Autodesk Fusion 360 part; units mm, degrees
(part 3 of 4)
extrude "Foro_PCB_reale_04" cut sketch "Schizzo5 (10)" along normal blind 2 bodies 26 in component "10_Modulo_cannone_reale_PCB_solenoide_canna"
ref_plane "Piano di lavoro2" through (0, 0, 85.5) normal (0, 0, 1) x (1, 0, 0) in component "10_Modulo_cannone_reale_PCB_solenoide_canna"
sketch "Schizzo6 (8)" plane through (0, 0, 85.5) normal (0, 0, 1) x (1, 0, 0) in component "10_Modulo_cannone_reale_PCB_solenoide_canna"
  line L0 (-10, 2.5) -> (10, 2.5)
  line L1 (10, 2.5) -> (10, 27.5)
  line L2 (10, 27.5) -> (-10, 27.5)
  line L3 (-10, 27.5) -> (-10, 2.5)
extrude "Estrusione_Appoggio_solenoide_su_PCB" add sketch "Schizzo6 (8)" along normal blind 1 separate body makes body 27 in component "10_Modulo_cannone_reale_PCB_solenoide_canna"
ref_plane "Piano di lavoro3" through (0, 2.5, 0) normal (0, 1, 0) x (0, 0, 1) in component "10_Modulo_cannone_reale_PCB_solenoide_canna"
sketch "Schizzo7 (8)" plane through (0, 2.5, 0) normal (0, 1, 0) x (1, 0, 0) in component "10_Modulo_cannone_reale_PCB_solenoide_canna"
  circle A0 centre (0, -96.5) radius 10
extrude "Estrusione_Corpo_solenoide_riferimento" add sketch "Schizzo7 (8)" along normal blind 25 separate body makes body 28 in component "10_Modulo_cannone_reale_PCB_solenoide_canna"
ref_plane "Piano di lavoro4" through (0, 2.5, 0) normal (0, 1, 0) x (0, 0, 1) in component "10_Modulo_cannone_reale_PCB_solenoide_canna"
sketch "Schizzo8 (8)" plane through (0, 2.5, 0) normal (0, 1, 0) x (1, 0, 0) in component "10_Modulo_cannone_reale_PCB_solenoide_canna"
  circle A0 centre (0, -96.5) radius 5
extrude "Passaggio_canna_nel_solenoide" cut sketch "Schizzo8 (8)" along normal blind 25 bodies 28 in component "10_Modulo_cannone_reale_PCB_solenoide_canna"
ref_plane "Piano di lavoro5" through (0, 27.5, 0) normal (0, 1, 0) x (0, 0, 1) in component "10_Modulo_cannone_reale_PCB_solenoide_canna"
sketch "Schizzo9 (8)" plane through (0, 27.5, 0) normal (0, 1, 0) x (1, 0, 0) in component "10_Modulo_cannone_reale_PCB_solenoide_canna"
  circle A0 centre (0, -96.5) radius 5
extrude "Estrusione_Canna_tubolare_esterna" add sketch "Schizzo9 (8)" along normal blind 46 separate body makes body 29 in component "10_Modulo_cannone_reale_PCB_solenoide_canna"
ref_plane "Piano di lavoro6" through (0, 27.5, 0) normal (0, 1, 0) x (0, 0, 1) in component "10_Modulo_cannone_reale_PCB_solenoide_canna"
sketch "Schizzo10 (8)" plane through (0, 27.5, 0) normal (0, 1, 0) x (1, 0, 0) in component "10_Modulo_cannone_reale_PCB_solenoide_canna"
  circle A0 centre (0, -96.5) radius 4
extrude "Foro_interno_canna_tubolare" cut sketch "Schizzo10 (8)" along normal blind 46 bodies 29 in component "10_Modulo_cannone_reale_PCB_solenoide_canna"
ref_plane "Piano di lavoro1" through (0, -38, 0) normal (0, 1, 0) x (0, 0, 1) in component "11_Guscio_fisso_posteriore_torretta_removibile"
sketch "Schizzo1 (23)" plane through (0, -38, 0) normal (0, 1, 0) x (1, 0, 0) in component "11_Guscio_fisso_posteriore_torretta_removibile"
  line L0 (-43, -49.5) -> (43, -49.5)
  line L1 (43, -49.5) -> (43, -102.5)
  line L2 (43, -102.5) -> (-43, -102.5)
  line L3 (-43, -102.5) -> (-43, -49.5)
extrude "Estrusione_Parete_posteriore_guscio_torretta" add sketch "Schizzo1 (23)" along normal blind 2.5 separate body makes body 30 in component "11_Guscio_fisso_posteriore_torretta_removibile"
ref_plane "Piano di lavoro2" through (-43, 0, 0) normal (1, 0, 0) x (0, 1, 0) in component "11_Guscio_fisso_posteriore_torretta_removibile"
sketch "Schizzo2 (21)" plane through (-43, 0, 0) normal (1, 0, 0) x (0, 0, -1) in component "11_Guscio_fisso_posteriore_torretta_removibile"
  line L0 (-49.5, -38) -> (-102.5, -38)
  line L1 (-102.5, -38) -> (-102.5, -27.8)
  line L2 (-102.5, -27.8) -> (-49.5, -27.8)
  line L3 (-49.5, -27.8) -> (-49.5, -38)
extrude "Estrusione_Fianco_cofano_Sinistra" add sketch "Schizzo2 (21)" along normal blind 2.5 bodies 30 in component "11_Guscio_fisso_posteriore_torretta_removibile"
ref_plane "Piano di lavoro3" through (40.5, 0, 0) normal (1, 0, 0) x (0, 1, 0) in component "11_Guscio_fisso_posteriore_torretta_removibile"
sketch "Schizzo3 (19)" plane through (40.5, 0, 0) normal (1, 0, 0) x (0, 0, -1) in component "11_Guscio_fisso_posteriore_torretta_removibile"
  line L0 (-49.5, -38) -> (-102.5, -38)
  line L1 (-102.5, -38) -> (-102.5, -27.8)
  line L2 (-102.5, -27.8) -> (-49.5, -27.8)
  line L3 (-49.5, -27.8) -> (-49.5, -38)
extrude "Estrusione_Fianco_cofano_Destra" add sketch "Schizzo3 (19)" along normal blind 2.5 bodies 30 in component "11_Guscio_fisso_posteriore_torretta_removibile"
ref_plane "Piano di lavoro4" through (0, 0, 100) normal (0, 0, 1) x (1, 0, 0) in component "11_Guscio_fisso_posteriore_torretta_removibile"
sketch "Schizzo4 (19)" plane through (0, 0, 100) normal (0, 0, 1) x (1, 0, 0) in component "11_Guscio_fisso_posteriore_torretta_removibile"
  line L0 (-43, -38) -> (43, -38)
  line L1 (43, -38) -> (43, -27.8)
  line L2 (43, -27.8) -> (-43, -27.8)
  line L3 (-43, -27.8) -> (-43, -38)
extrude "Estrusione_Tetto_cofano_posteriore" add sketch "Schizzo4 (19)" along normal blind 2.5 bodies 30 in component "11_Guscio_fisso_posteriore_torretta_removibile"
ref_plane "Piano di lavoro5" through (-43, 0, 0) normal (1, 0, 0) x (0, 1, 0) in component "11_Guscio_fisso_posteriore_torretta_removibile"
sketch "Schizzo5 (11)" plane through (-43, 0, 0) normal (1, 0, 0) x (0, 0, -1) in component "11_Guscio_fisso_posteriore_torretta_removibile"
  circle A0 centre (-54.5, -30.3) radius 1.35
extrude "Foro_M2_5_cofano_Sinistra_01" cut sketch "Schizzo5 (11)" along normal blind 2.5 bodies 30 in component "11_Guscio_fisso_posteriore_torretta_removibile"
ref_plane "Piano di lavoro27" through (-40, 0, 0) normal (1, 0, 0) x (0, 1, 0) in component "04_Torretta_parte_fissa_azimut"
sketch "Schizzo41 (2)" plane through (-40, 0, 0) normal (1, 0, 0) x (0, 0, -1) in component "04_Torretta_parte_fissa_azimut"
  circle A0 centre (-54.5, -30.3) radius 1.1
extrude "Preforo_M2_5_cofano_telaio_Sinistra_01" cut sketch "Schizzo41 (2)" along normal blind 4 bodies 14 in component "04_Torretta_parte_fissa_azimut"
ref_plane "Piano di lavoro6" through (-43, 0, 0) normal (1, 0, 0) x (0, 1, 0) in component "11_Guscio_fisso_posteriore_torretta_removibile"
sketch "Schizzo6 (9)" plane through (-43, 0, 0) normal (1, 0, 0) x (0, 0, -1) in component "11_Guscio_fisso_posteriore_torretta_removibile"
  circle A0 centre (-94.5, -30.3) radius 1.35
extrude "Foro_M2_5_cofano_Sinistra_02" cut sketch "Schizzo6 (9)" along normal blind 2.5 bodies 30 in component "11_Guscio_fisso_posteriore_torretta_removibile"
ref_plane "Piano di lavoro28" through (-40, 0, 0) normal (1, 0, 0) x (0, 1, 0) in component "04_Torretta_parte_fissa_azimut"
sketch "Schizzo42 (2)" plane through (-40, 0, 0) normal (1, 0, 0) x (0, 0, -1) in component "04_Torretta_parte_fissa_azimut"
  circle A0 centre (-94.5, -30.3) radius 1.1
extrude "Preforo_M2_5_cofano_telaio_Sinistra_02" cut sketch "Schizzo42 (2)" along normal blind 4 bodies 14 in component "04_Torretta_parte_fissa_azimut"
ref_plane "Piano di lavoro7" through (40.5, 0, 0) normal (1, 0, 0) x (0, 1, 0) in component "11_Guscio_fisso_posteriore_torretta_removibile"
sketch "Schizzo7 (9)" plane through (40.5, 0, 0) normal (1, 0, 0) x (0, 0, -1) in component "11_Guscio_fisso_posteriore_torretta_removibile"
  circle A0 centre (-54.5, -30.3) radius 1.35
extrude "Foro_M2_5_cofano_Destra_01" cut sketch "Schizzo7 (9)" along normal blind 2.5 bodies 30 in component "11_Guscio_fisso_posteriore_torretta_removibile"
ref_plane "Piano di lavoro29" through (36, 0, 0) normal (1, 0, 0) x (0, 1, 0) in component "04_Torretta_parte_fissa_azimut"
sketch "Schizzo43 (2)" plane through (36, 0, 0) normal (1, 0, 0) x (0, 0, -1) in component "04_Torretta_parte_fissa_azimut"
  circle A0 centre (-54.5, -30.3) radius 1.1
extrude "Preforo_M2_5_cofano_telaio_Destra_01" cut sketch "Schizzo43 (2)" along normal blind 4 bodies 14 in component "04_Torretta_parte_fissa_azimut"
ref_plane "Piano di lavoro8" through (40.5, 0, 0) normal (1, 0, 0) x (0, 1, 0) in component "11_Guscio_fisso_posteriore_torretta_removibile"
sketch "Schizzo8 (9)" plane through (40.5, 0, 0) normal (1, 0, 0) x (0, 0, -1) in component "11_Guscio_fisso_posteriore_torretta_removibile"
  circle A0 centre (-94.5, -30.3) radius 1.35
extrude "Foro_M2_5_cofano_Destra_02" cut sketch "Schizzo8 (9)" along normal blind 2.5 bodies 30 in component "11_Guscio_fisso_posteriore_torretta_removibile"
ref_plane "Piano di lavoro30" through (36, 0, 0) normal (1, 0, 0) x (0, 1, 0) in component "04_Torretta_parte_fissa_azimut"
sketch "Schizzo44" plane through (36, 0, 0) normal (1, 0, 0) x (0, 0, -1) in component "04_Torretta_parte_fissa_azimut"
  circle A0 centre (-94.5, -30.3) radius 1.1
extrude "Preforo_M2_5_cofano_telaio_Destra_02" cut sketch "Schizzo44" along normal blind 4 bodies 14 in component "04_Torretta_parte_fissa_azimut"
ref_plane "Piano di lavoro1" through (-66.5, 0, 0) normal (1, 0, 0) x (0, 1, 0) in component "12_Carter_SG90_Sinistro_removibile"
sketch "Schizzo1 (24)" plane through (-66.5, 0, 0) normal (1, 0, 0) x (0, 0, -1) in component "12_Carter_SG90_Sinistro_removibile"
  line L0 (-71.9, -27.8) -> (-93.6, -27.8)
  line L1 (-93.6, -27.8) -> (-93.6, 16.5)
  line L2 (-93.6, 16.5) -> (-71.9, 16.5)
  line L3 (-71.9, 16.5) -> (-71.9, -27.8)
extrude "Estrusione_Parete_esterna_carter_Sinistro" add sketch "Schizzo1 (24)" along normal blind 2.5 separate body makes body 31 in component "12_Carter_SG90_Sinistro_removibile"
ref_plane "Piano di lavoro2" through (0, -27.8, 0) normal (0, 1, 0) x (0, 0, 1) in component "12_Carter_SG90_Sinistro_removibile"
sketch "Schizzo2 (22)" plane through (0, -27.8, 0) normal (0, 1, 0) x (1, 0, 0) in component "12_Carter_SG90_Sinistro_removibile"
  line L0 (-66.5, -71.9) -> (-40.5, -71.9)
  line L1 (-40.5, -71.9) -> (-40.5, -93.6)
  line L2 (-40.5, -93.6) -> (-66.5, -93.6)
  line L3 (-66.5, -93.6) -> (-66.5, -71.9)
extrude "Estrusione_Parete_Posteriore_carter_Sinistro" add sketch "Schizzo2 (22)" along normal blind 2.5 bodies 31 in component "12_Carter_SG90_Sinistro_removibile"
ref_plane "Piano di lavoro3" through (0, 14, 0) normal (0, 1, 0) x (0, 0, 1) in component "12_Carter_SG90_Sinistro_removibile"
sketch "Schizzo3 (20)" plane through (0, 14, 0) normal (0, 1, 0) x (1, 0, 0) in component "12_Carter_SG90_Sinistro_removibile"
  line L0 (-66.5, -71.9) -> (-40.5, -71.9)
  line L1 (-40.5, -71.9) -> (-40.5, -93.6)
  line L2 (-40.5, -93.6) -> (-66.5, -93.6)
  line L3 (-66.5, -93.6) -> (-66.5, -71.9)
extrude "Estrusione_Parete_Anteriore_carter_Sinistro" add sketch "Schizzo3 (20)" along normal blind 2.5 bodies 31 in component "12_Carter_SG90_Sinistro_removibile"
ref_plane "Piano di lavoro4" through (0, 0, 91.1) normal (0, 0, 1) x (1, 0, 0) in component "12_Carter_SG90_Sinistro_removibile"
sketch "Schizzo4 (20)" plane through (0, 0, 91.1) normal (0, 0, 1) x (1, 0, 0) in component "12_Carter_SG90_Sinistro_removibile"
  line L0 (-66.5, -27.8) -> (-40.5, -27.8)
  line L1 (-40.5, -27.8) -> (-40.5, 16.5)
  line L2 (-40.5, 16.5) -> (-66.5, 16.5)
  line L3 (-66.5, 16.5) -> (-66.5, -27.8)
extrude "Estrusione_Tetto_carter_Sinistro" add sketch "Schizzo4 (20)" along normal blind 2.5 bodies 31 in component "12_Carter_SG90_Sinistro_removibile"
ref_plane "Piano di lavoro5" through (-66.5, 0, 0) normal (1, 0, 0) x (0, 1, 0) in component "12_Carter_SG90_Sinistro_removibile"
sketch "Schizzo5 (12)" plane through (-66.5, 0, 0) normal (1, 0, 0) x (0, 0, -1) in component "12_Carter_SG90_Sinistro_removibile"
  circle A0 centre (-81.5, -23.55) radius 1.35
extrude "Foro_M2_5_carter_Sinistro_01" cut sketch "Schizzo5 (12)" along normal blind 2.5 bodies 31 in component "12_Carter_SG90_Sinistro_removibile"
ref_plane "Piano di lavoro6" through (-66.5, 0, 0) normal (1, 0, 0) x (0, 1, 0) in component "12_Carter_SG90_Sinistro_removibile"
sketch "Schizzo6 (10)" plane through (-66.5, 0, 0) normal (1, 0, 0) x (0, 0, -1) in component "12_Carter_SG90_Sinistro_removibile"
  circle A0 centre (-81.5, 12.25) radius 1.35
extrude "Foro_M2_5_carter_Sinistro_02" cut sketch "Schizzo6 (10)" along normal blind 2.5 bodies 31 in component "12_Carter_SG90_Sinistro_removibile"
ref_plane "Piano di lavoro1" through (64, 0, 0) normal (1, 0, 0) x (0, 1, 0) in component "13_Carter_SG90_Destro_removibile"
sketch "Schizzo1 (25)" plane through (64, 0, 0) normal (1, 0, 0) x (0, 0, -1) in component "13_Carter_SG90_Destro_removibile"
  line L0 (-71.9, -27.8) -> (-93.6, -27.8)
  line L1 (-93.6, -27.8) -> (-93.6, 16.5)
  line L2 (-93.6, 16.5) -> (-71.9, 16.5)
  line L3 (-71.9, 16.5) -> (-71.9, -27.8)
extrude "Estrusione_Parete_esterna_carter_Destro" add sketch "Schizzo1 (25)" along normal blind 2.5 separate body makes body 32 in component "13_Carter_SG90_Destro_removibile"
ref_plane "Piano di lavoro2" through (0, -27.8, 0) normal (0, 1, 0) x (0, 0, 1) in component "13_Carter_SG90_Destro_removibile"
sketch "Schizzo2 (23)" plane through (0, -27.8, 0) normal (0, 1, 0) x (1, 0, 0) in component "13_Carter_SG90_Destro_removibile"
  line L0 (40.5, -71.9) -> (66.5, -71.9)
  line L1 (66.5, -71.9) -> (66.5, -93.6)
  line L2 (66.5, -93.6) -> (40.5, -93.6)
  line L3 (40.5, -93.6) -> (40.5, -71.9)
extrude "Estrusione_Parete_Posteriore_carter_Destro" add sketch "Schizzo2 (23)" along normal blind 2.5 bodies 32 in component "13_Carter_SG90_Destro_removibile"
ref_plane "Piano di lavoro3" through (0, 14, 0) normal (0, 1, 0) x (0, 0, 1) in component "13_Carter_SG90_Destro_removibile"
sketch "Schizzo3 (21)" plane through (0, 14, 0) normal (0, 1, 0) x (1, 0, 0) in component "13_Carter_SG90_Destro_removibile"
  line L0 (40.5, -71.9) -> (66.5, -71.9)
  line L1 (66.5, -71.9) -> (66.5, -93.6)
  line L2 (66.5, -93.6) -> (40.5, -93.6)
  line L3 (40.5, -93.6) -> (40.5, -71.9)
extrude "Estrusione_Parete_Anteriore_carter_Destro" add sketch "Schizzo3 (21)" along normal blind 2.5 bodies 32 in component "13_Carter_SG90_Destro_removibile"
ref_plane "Piano di lavoro4" through (0, 0, 91.1) normal (0, 0, 1) x (1, 0, 0) in component "13_Carter_SG90_Destro_removibile"
sketch "Schizzo4 (21)" plane through (0, 0, 91.1) normal (0, 0, 1) x (1, 0, 0) in component "13_Carter_SG90_Destro_removibile"
  line L0 (40.5, -27.8) -> (66.5, -27.8)
  line L1 (66.5, -27.8) -> (66.5, 16.5)
  line L2 (66.5, 16.5) -> (40.5, 16.5)
  line L3 (40.5, 16.5) -> (40.5, -27.8)
extrude "Estrusione_Tetto_carter_Destro" add sketch "Schizzo4 (21)" along normal blind 2.5 bodies 32 in component "13_Carter_SG90_Destro_removibile"
ref_plane "Piano di lavoro5" through (64, 0, 0) normal (1, 0, 0) x (0, 1, 0) in component "13_Carter_SG90_Destro_removibile"
sketch "Schizzo5 (13)" plane through (64, 0, 0) normal (1, 0, 0) x (0, 0, -1) in component "13_Carter_SG90_Destro_removibile"
  circle A0 centre (-81.5, -23.55) radius 1.35
extrude "Foro_M2_5_carter_Destro_01" cut sketch "Schizzo5 (13)" along normal blind 2.5 bodies 32 in component "13_Carter_SG90_Destro_removibile"
ref_plane "Piano di lavoro6" through (64, 0, 0) normal (1, 0, 0) x (0, 1, 0) in component "13_Carter_SG90_Destro_removibile"
sketch "Schizzo6 (11)" plane through (64, 0, 0) normal (1, 0, 0) x (0, 0, -1) in component "13_Carter_SG90_Destro_removibile"
  circle A0 centre (-81.5, 12.25) radius 1.35
extrude "Foro_M2_5_carter_Destro_02" cut sketch "Schizzo6 (11)" along normal blind 2.5 bodies 32 in component "13_Carter_SG90_Destro_removibile"
ref_plane "Piano di lavoro1" through (0, 0, 83.5) normal (0, 0, 1) x (1, 0, 0) in component "14_Guscio_mobile_cannone_removibile"
sketch "Schizzo1 (26)" plane through (0, 0, 83.5) normal (0, 0, 1) x (1, 0, 0) in component "14_Guscio_mobile_cannone_removibile"
  line L0 (-28, -13) -> (-25.5, -13)
  line L1 (-25.5, -13) -> (-25.5, 43)
  line L2 (-25.5, 43) -> (-28, 43)
  line L3 (-28, 43) -> (-28, -13)
extrude "Estrusione_Parete_mobile_Ovest" add sketch "Schizzo1 (26)" along normal blind 26 separate body makes body 33 in component "14_Guscio_mobile_cannone_removibile"
sketch "Schizzo2 (24)" plane through (0, 0, 83.5) normal (0, 0, 1) x (1, 0, 0) in component "14_Guscio_mobile_cannone_removibile"
  line L0 (-28, -13) -> (28, -13)
  line L1 (28, -13) -> (28, -10.5)
  line L2 (28, -10.5) -> (-28, -10.5)
  line L3 (-28, -10.5) -> (-28, -13)
extrude "Estrusione_Parete_mobile_Posteriore" add sketch "Schizzo2 (24)" along normal blind 26 bodies 33 in component "14_Guscio_mobile_cannone_removibile"
sketch "Schizzo3 (22)" plane through (0, 0, 83.5) normal (0, 0, 1) x (1, 0, 0) in component "14_Guscio_mobile_cannone_removibile"
  line L0 (25.5, -13) -> (28, -13)
  line L1 (28, -13) -> (28, 43)
  line L2 (28, 43) -> (25.5, 43)
  line L3 (25.5, 43) -> (25.5, -13)
extrude "Estrusione_Parete_mobile_Est" add sketch "Schizzo3 (22)" along normal blind 26 bodies 33 in component "14_Guscio_mobile_cannone_removibile"
ref_plane "Piano di lavoro2" through (-28, 0, 0) normal (1, 0, 0) x (0, 1, 0) in component "14_Guscio_mobile_cannone_removibile"
sketch "Schizzo4 (22)" plane through (-28, 0, 0) normal (1, 0, 0) x (0, 0, -1) in component "14_Guscio_mobile_cannone_removibile"
  circle A0 centre (-81.5, 0) radius 17.5
extrude "Scasso_guancia_elevazione_Ovest" cut sketch "Schizzo4 (22)" along normal blind 2.5 bodies 17 in component "09_Torretta_parte_mobile_elevazione"
extrude "Estrusione6" cut sketch "Schizzo4 (22)" along normal blind 2.5 bodies 22 makes body 34 at (-31, -1.093, 68.5819) in component "09A_Guancia_cornetto_Sinistra_regolabile"
extrude "Estrusione4'" cut sketch "Schizzo4 (22)" along normal blind 2.5 bodies 33 in component "14_Guscio_mobile_cannone_removibile"
ref_plane "Piano di lavoro3" through (25.5, 0, 0) normal (1, 0, 0) x (0, 1, 0) in component "14_Guscio_mobile_cannone_removibile"
sketch "Schizzo5 (14)" plane through (25.5, 0, 0) normal (1, 0, 0) x (0, 0, -1) in component "14_Guscio_mobile_cannone_removibile"
  circle A0 centre (-81.5, 0) radius 17.5
extrude "Scasso_guancia_elevazione_Est" cut sketch "Schizzo5 (14)" along normal blind 2.5 bodies 17 in component "09_Torretta_parte_mobile_elevazione"
extrude "Estrusione6'" cut sketch "Schizzo5 (14)" along normal blind 2.5 bodies 24 makes body 35 at (23.3333, -2.85, 79.5) in component "09B_Guancia_cornetto_Destra_regolabile"
extrude "Estrusione5" cut sketch "Schizzo5 (14)" along normal blind 2.5 bodies 33 in component "14_Guscio_mobile_cannone_removibile"
ref_plane "Piano di lavoro4" through (0, 0, 107) normal (0, 0, 1) x (1, 0, 0) in component "14_Guscio_mobile_cannone_removibile"
sketch "Schizzo6 (12)" plane through (0, 0, 107) normal (0, 0, 1) x (1, 0, 0) in component "14_Guscio_mobile_cannone_removibile"
  line L0 (-28, -13) -> (28, -13)
  line L1 (28, -13) -> (28, 43)
  line L2 (28, 43) -> (-28, 43)
  line L3 (-28, 43) -> (-28, -13)
extrude "Estrusione_Tetto_guscio_mobile_cannone" add sketch "Schizzo6 (12)" along normal blind 2.5 bodies 33 in component "14_Guscio_mobile_cannone_removibile"
ref_plane "Piano di lavoro5" through (0, 0, 106.2) normal (0, 0, 1) x (1, 0, 0) in component "14_Guscio_mobile_cannone_removibile"
sketch "Schizzo7 (10)" plane through (0, 0, 106.2) normal (0, 0, 1) x (1, 0, 0) in component "14_Guscio_mobile_cannone_removibile"
  line L0 (-15, -13) -> (-7, -13)
  line L1 (-7, -13) -> (-7, 2)
  line L2 (-7, 2) -> (-15, 2)
  line L3 (-15, 2) -> (-15, -13)
extrude "Estrusione_Longherone_rinforzo_tasca_culatta_Ovest" add sketch "Schizzo7 (10)" along normal blind 1 bodies 33 in component "14_Guscio_mobile_cannone_removibile"
sketch "Schizzo8 (10)" plane through (0, 0, 106.2) normal (0, 0, 1) x (1, 0, 0) in component "14_Guscio_mobile_cannone_removibile"
  line L0 (7, -13) -> (15, -13)
  line L1 (15, -13) -> (15, 2)
  line L2 (15, 2) -> (7, 2)
  line L3 (7, 2) -> (7, -13)
extrude "Estrusione_Longherone_rinforzo_tasca_culatta_Est" add sketch "Schizzo8 (10)" along normal blind 1 bodies 33 in component "14_Guscio_mobile_cannone_removibile"
sketch "Schizzo9 (9)" plane through (0, 0, 106.2) normal (0, 0, 1) x (1, 0, 0) in component "14_Guscio_mobile_cannone_removibile"
  line L0 (-15, -1) -> (15, -1)
  line L1 (15, -1) -> (15, 2)
  line L2 (15, 2) -> (-15, 2)
  line L3 (-15, 2) -> (-15, -1)
extrude "Estrusione_Traversa_anteriore_rinforzo_tasca_culatta" add sketch "Schizzo9 (9)" along normal blind 1 bodies 33 in component "14_Guscio_mobile_cannone_removibile"
ref_plane "Piano di lavoro6" through (0, -13, 0) normal (0, 1, 0) x (0, 0, 1) in component "14_Guscio_mobile_cannone_removibile"
sketch "Schizzo10 (9)" plane through (0, -13, 0) normal (0, 1, 0) x (1, 0, 0) in component "14_Guscio_mobile_cannone_removibile"
  line L0 (-7, -90.5) -> (7, -90.5)
  line L1 (7, -90.5) -> (7, -109.5)
  line L2 (7, -109.5) -> (-7, -109.5)
  line L3 (-7, -109.5) -> (-7, -90.5)
extrude "Finestra_posteriore_culatta_manuale" cut sketch "Schizzo10 (9)" along normal blind 2.5 bodies 33 in component "14_Guscio_mobile_cannone_removibile"
sketch "Schizzo11 (8)" plane through (0, 0, 107) normal (0, 0, 1) x (1, 0, 0) in component "14_Guscio_mobile_cannone_removibile"
  line L0 (-7, -13) -> (7, -13)
  line L1 (7, -13) -> (7, -1)
  line L2 (7, -1) -> (-7, -1)
  line L3 (-7, -1) -> (-7, -13)
extrude "Asola_tetto_accesso_culatta_manuale" cut sketch "Schizzo11 (8)" along normal blind 2.5 bodies 33 in component "14_Guscio_mobile_cannone_removibile"
ref_plane "Piano di lavoro7" through (0, 0, 107.5) normal (0, 0, 1) x (1, 0, 0) in component "14_Guscio_mobile_cannone_removibile"
sketch "Schizzo12 (7)" plane through (0, 0, 107.5) normal (0, 0, 1) x (1, 0, 0) in component "14_Guscio_mobile_cannone_removibile"
  line L0 (-15, -13) -> (15, -13)
  line L1 (15, -13) -> (15, 2)
  line L2 (15, 2) -> (-15, 2)
  line L3 (-15, 2) -> (-15, -13)
extrude "Tasca_coperchio_culatta_a_filo" cut sketch "Schizzo12 (7)" along normal blind 2 bodies 33 in component "14_Guscio_mobile_cannone_removibile"
ref_plane "Piano di lavoro8" through (0, -6, 0) normal (0, 1, 0) x (0, 0, 1) in component "14_Guscio_mobile_cannone_removibile"
sketch "Schizzo13 (7)" plane through (0, -6, 0) normal (0, 1, 0) x (1, 0, 0) in component "14_Guscio_mobile_cannone_removibile"
  circle A0 centre (0, -96.5) radius 5.5
extrude "Estrusione_Guida_interna_culatta_manuale" add sketch "Schizzo13 (7)" along normal blind 8 separate body makes body 36 in component "14_Guscio_mobile_cannone_removibile"
ref_plane "Piano di lavoro9" through (0, -6, 0) normal (0, 1, 0) x (0, 0, 1) in component "14_Guscio_mobile_cannone_removibile"
sketch "Schizzo14 (6)" plane through (0, -6, 0) normal (0, 1, 0) x (1, 0, 0) in component "14_Guscio_mobile_cannone_removibile"
  circle A0 centre (0, -96.5) radius 4
extrude "Foro_coassiale_guida_culatta_manuale" cut sketch "Schizzo14 (6)" along normal blind 8 bodies 36 in component "14_Guscio_mobile_cannone_removibile"
ref_plane "Piano di lavoro10" through (0, 0, 100.8) normal (0, 0, 1) x (1, 0, 0) in component "14_Guscio_mobile_cannone_removibile"
sketch "Schizzo15 (6)" plane through (0, 0, 100.8) normal (0, 0, 1) x (1, 0, 0) in component "14_Guscio_mobile_cannone_removibile"
  line L0 (-2, -6) -> (2, -6)
  line L1 (2, -6) -> (2, 2)
  line L2 (2, 2) -> (-2, 2)
  line L3 (-2, 2) -> (-2, -6)
extrude "Estrusione_Nervatura_tetto_guida_culatta" add sketch "Schizzo15 (6)" along normal blind 6.4 bodies 33 36 in component "14_Guscio_mobile_cannone_removibile"
ref_plane "Piano di lavoro11" through (0, 0, 103) normal (0, 0, 1) x (1, 0, 0) in component "14_Guscio_mobile_cannone_removibile"
sketch "Schizzo16 (6)" plane through (0, 0, 103) normal (0, 0, 1) x (1, 0, 0) in component "14_Guscio_mobile_cannone_removibile"
  circle A0 centre (-10.75, -4) radius 3
extrude "Estrusione_Boss_M2_5_coperchio_culatta_01" add sketch "Schizzo16 (6)" along normal blind 4.2 bodies 33 in component "14_Guscio_mobile_cannone_removibile"
sketch "Schizzo17 (5)" plane through (0, 0, 103) normal (0, 0, 1) x (1, 0, 0) in component "14_Guscio_mobile_cannone_removibile"
  circle A0 centre (-10.75, -4) radius 1.1
extrude "Preforo_M2_5_coperchio_culatta_01" cut sketch "Schizzo17 (5)" along normal blind 4.6 bodies 33 in component "14_Guscio_mobile_cannone_removibile"
sketch "Schizzo18 (5)" plane through (0, 0, 103) normal (0, 0, 1) x (1, 0, 0) in component "14_Guscio_mobile_cannone_removibile"
  circle A0 centre (10.75, -4) radius 3
extrude "Estrusione_Boss_M2_5_coperchio_culatta_02" add sketch "Schizzo18 (5)" along normal blind 4.2 bodies 33 in component "14_Guscio_mobile_cannone_removibile"
sketch "Schizzo19 (4)" plane through (0, 0, 103) normal (0, 0, 1) x (1, 0, 0) in component "14_Guscio_mobile_cannone_removibile"
  circle A0 centre (10.75, -4) radius 1.1
extrude "Preforo_M2_5_coperchio_culatta_02" cut sketch "Schizzo19 (4)" along normal blind 4.6 bodies 33 in component "14_Guscio_mobile_cannone_removibile"
sketch "Schizzo20 (4)" plane through (0, 0, 83.5) normal (0, 0, 1) x (1, 0, 0) in component "14_Guscio_mobile_cannone_removibile"
  line L0 (-28, 40.5) -> (-5.5, 40.5)
  line L1 (-5.5, 40.5) -> (-5.5, 43)
  line L2 (-5.5, 43) -> (-28, 43)
  line L3 (-28, 43) -> (-28, 40.5)
extrude "Estrusione_Parete_mobile_Anteriore_Ovest" add sketch "Schizzo20 (4)" along normal blind 26 bodies 33 in component "14_Guscio_mobile_cannone_removibile"
sketch "Schizzo21 (4)" plane through (0, 0, 83.5) normal (0, 0, 1) x (1, 0, 0) in component "14_Guscio_mobile_cannone_removibile"
  line L0 (5.5, 40.5) -> (28, 40.5)
  line L1 (28, 40.5) -> (28, 43)
  line L2 (28, 43) -> (5.5, 43)
  line L3 (5.5, 43) -> (5.5, 40.5)
extrude "Estrusione_Parete_mobile_Anteriore_Est" add sketch "Schizzo21 (4)" along normal blind 26 bodies 33 in component "14_Guscio_mobile_cannone_removibile"
ref_plane "Piano di lavoro12" through (0, 0, 102) normal (0, 0, 1) x (1, 0, 0) in component "14_Guscio_mobile_cannone_removibile"
sketch "Schizzo22 (4)" plane through (0, 0, 102) normal (0, 0, 1) x (1, 0, 0) in component "14_Guscio_mobile_cannone_removibile"
  line L0 (-5.5, 40.5) -> (5.5, 40.5)
  line L1 (5.5, 40.5) -> (5.5, 43)
  line L2 (5.5, 43) -> (-5.5, 43)
  line L3 (-5.5, 43) -> (-5.5, 40.5)
extrude "Estrusione_Ponte_superiore_cava_U_canna" add sketch "Schizzo22 (4)" along normal blind 7.5 bodies 33 in component "14_Guscio_mobile_cannone_removibile"
ref_plane "Piano di lavoro13" through (0, -13, 0) normal (0, 1, 0) x (0, 0, 1) in component "14_Guscio_mobile_cannone_removibile"
sketch "Schizzo23 (3)" plane through (0, -13, 0) normal (0, 1, 0) x (1, 0, 0) in component "14_Guscio_mobile_cannone_removibile"
  line L0 (-3, -83.5) -> (3, -83.5)
  line L1 (3, -83.5) -> (3, -87.5)
  line L2 (3, -87.5) -> (-3, -87.5)
  line L3 (-3, -87.5) -> (-3, -83.5)
extrude "Tacca_posteriore_cavo_cannone_aperta_inferiormente" cut sketch "Schizzo23 (3)" along normal blind 2.5 bodies 33 in component "14_Guscio_mobile_cannone_removibile"
ref_plane "Piano di lavoro14" through (0, 0, 85.5) normal (0, 0, 1) x (1, 0, 0) in component "14_Guscio_mobile_cannone_removibile"
sketch "Schizzo24 (3)" plane through (0, 0, 85.5) normal (0, 0, 1) x (1, 0, 0) in component "14_Guscio_mobile_cannone_removibile"
  circle A0 centre (-20, -5) radius 5
extrude "Estrusione_Colonna_M3_guscio_mobile_01" add sketch "Schizzo24 (3)" along normal blind 21.7 bodies 33 in component "14_Guscio_mobile_cannone_removibile"
sketch "Schizzo25 (3)" plane through (0, 0, 85.5) normal (0, 0, 1) x (1, 0, 0) in component "14_Guscio_mobile_cannone_removibile"
  circle A0 centre (-20, -5) radius 1.75
extrude "Foro_M3_guscio_mobile_01" cut sketch "Schizzo25 (3)" along normal blind 24 bodies 33 in component "14_Guscio_mobile_cannone_removibile"
sketch "Schizzo26 (3)" plane through (0, 0, 85.5) normal (0, 0, 1) x (1, 0, 0) in component "14_Guscio_mobile_cannone_removibile"
  circle A0 centre (20, -5) radius 5
extrude "Estrusione_Colonna_M3_guscio_mobile_02" add sketch "Schizzo26 (3)" along normal blind 21.7 bodies 33 in component "14_Guscio_mobile_cannone_removibile"
sketch "Schizzo27 (3)" plane through (0, 0, 85.5) normal (0, 0, 1) x (1, 0, 0) in component "14_Guscio_mobile_cannone_removibile"
  circle A0 centre (20, -5) radius 1.75
extrude "Foro_M3_guscio_mobile_02" cut sketch "Schizzo27 (3)" along normal blind 24 bodies 33 in component "14_Guscio_mobile_cannone_removibile"
sketch "Schizzo28 (3)" plane through (0, 0, 85.5) normal (0, 0, 1) x (1, 0, 0) in component "14_Guscio_mobile_cannone_removibile"
  circle A0 centre (-20, 35) radius 5
extrude "Estrusione_Colonna_M3_guscio_mobile_03" add sketch "Schizzo28 (3)" along normal blind 21.7 bodies 33 in component "14_Guscio_mobile_cannone_removibile"
sketch "Schizzo29 (3)" plane through (0, 0, 85.5) normal (0, 0, 1) x (1, 0, 0) in component "14_Guscio_mobile_cannone_removibile"
  circle A0 centre (-20, 35) radius 1.75
extrude "Foro_M3_guscio_mobile_03" cut sketch "Schizzo29 (3)" along normal blind 24 bodies 33 in component "14_Guscio_mobile_cannone_removibile"
sketch "Schizzo30 (3)" plane through (0, 0, 85.5) normal (0, 0, 1) x (1, 0, 0) in component "14_Guscio_mobile_cannone_removibile"
  circle A0 centre (20, 35) radius 5
extrude "Estrusione_Colonna_M3_guscio_mobile_04" add sketch "Schizzo30 (3)" along normal blind 21.7 bodies 33 in component "14_Guscio_mobile_cannone_removibile"
sketch "Schizzo31 (3)" plane through (0, 0, 85.5) normal (0, 0, 1) x (1, 0, 0) in component "14_Guscio_mobile_cannone_removibile"
  circle A0 centre (20, 35) radius 1.75
extrude "Foro_M3_guscio_mobile_04" cut sketch "Schizzo31 (3)" along normal blind 24 bodies 33 in component "14_Guscio_mobile_cannone_removibile"
ref_plane "Piano di lavoro1" through (0, 0, 107.5) normal (0, 0, 1) x (1, 0, 0) in component "15_Coperchio_culatta_L_removibile_M2_5"
sketch "Schizzo1 (27)" plane through (0, 0, 107.5) normal (0, 0, 1) x (1, 0, 0) in component "15_Coperchio_culatta_L_removibile_M2_5"
  line L0 (-14.7, -12.7) -> (14.7, -12.7)
  line L1 (14.7, -12.7) -> (14.7, 1.7)
  line L2 (14.7, 1.7) -> (-14.7, 1.7)
  line L3 (-14.7, 1.7) -> (-14.7, -12.7)
extrude "Estrusione_Piastra_superiore_coperchio_culatta_a_filo" add sketch "Schizzo1 (27)" along normal blind 1.8 separate body makes body 37 in component "15_Coperchio_culatta_L_removibile_M2_5"
ref_plane "Piano di lavoro2" through (0, -12.7, 0) normal (0, 1, 0) x (0, 0, 1) in component "15_Coperchio_culatta_L_removibile_M2_5"
sketch "Schizzo2 (25)" plane through (0, -12.7, 0) normal (0, 1, 0) x (1, 0, 0) in component "15_Coperchio_culatta_L_removibile_M2_5"
  line L0 (-6.7, -90.8) -> (6.7, -90.8)
  line L1 (6.7, -90.8) -> (6.7, -109.2)
  line L2 (6.7, -109.2) -> (-6.7, -109.2)
  line L3 (-6.7, -109.2) -> (-6.7, -90.8)
extrude "Estrusione_Piastra_posteriore_coperchio_culatta" add sketch "Schizzo2 (25)" along normal blind 1.9 bodies 37 in component "15_Coperchio_culatta_L_removibile_M2_5"
ref_plane "Piano di lavoro3" through (0, 0, 108.1) normal (0, 0, 1) x (1, 0, 0) in component "15_Coperchio_culatta_L_removibile_M2_5"
ref_plane "Piano di lavoro4" through (0, 0, 109.3) normal (0, 0, 1) x (1, 0, 0) in component "15_Coperchio_culatta_L_removibile_M2_5"
sketch "Schizzo3 (23)" plane through (0, 0, 107.5) normal (0, 0, 1) x (1, 0, 0) in component "15_Coperchio_culatta_L_removibile_M2_5"
  circle A0 centre (-10.75, -4) radius 1.35
extrude "Foro_M2_5_coperchio_culatta_01" cut sketch "Schizzo3 (23)" along normal blind 1.8 bodies 37 in component "15_Coperchio_culatta_L_removibile_M2_5"
sketch "Schizzo4 (23)" plane through (0, 0, 108.1) normal (0, 0, 1) x (1, 0, 0) in component "15_Coperchio_culatta_L_removibile_M2_5"
  circle A0 centre (-10.75, -4) radius 1.35
sketch "Schizzo5 (15)" plane through (0, 0, 109.3) normal (0, 0, 1) x (1, 0, 0) in component "15_Coperchio_culatta_L_removibile_M2_5"
  circle A0 centre (-10.75, -4) radius 2.5
loft "Svasatura_M2_5_coperchio_culatta_01" cut profiles "Schizzo4 (23)", "Schizzo5 (15)" section 1 section 2 bodies 37 in component "15_Coperchio_culatta_L_removibile_M2_5"
sketch "Schizzo6 (13)" plane through (0, 0, 107.5) normal (0, 0, 1) x (1, 0, 0) in component "15_Coperchio_culatta_L_removibile_M2_5"
  circle A0 centre (10.75, -4) radius 1.35
extrude "Foro_M2_5_coperchio_culatta_02" cut sketch "Schizzo6 (13)" along normal blind 1.8 bodies 37 in component "15_Coperchio_culatta_L_removibile_M2_5"
sketch "Schizzo7 (11)" plane through (0, 0, 108.1) normal (0, 0, 1) x (1, 0, 0) in component "15_Coperchio_culatta_L_removibile_M2_5"
  circle A0 centre (10.75, -4) radius 1.35
sketch "Schizzo8 (11)" plane through (0, 0, 109.3) normal (0, 0, 1) x (1, 0, 0) in component "15_Coperchio_culatta_L_removibile_M2_5"
  circle A0 centre (10.75, -4) radius 2.5
loft "Svasatura_M2_5_coperchio_culatta_02" cut profiles "Schizzo7 (11)", "Schizzo8 (11)" section 1 section 2 bodies 37 in component "15_Coperchio_culatta_L_removibile_M2_5"
sketch "Schizzo1 (28)" plane through (0, 0, 0) normal (0, 1, 0) x (1, 0, 0) in component "06_Sottoassieme_coperchio_stepper_torretta"
  line L0 (0, -20) -> (0, 20)
ref_plane "Piano di lavoro1" through (0, 0, 81.5) normal (0, 0, 1) x (1, 0, 0) in component "06_Sottoassieme_coperchio_stepper_torretta"
sketch "Schizzo2 (26)" plane through (0, 0, 81.5) normal (0, 0, 1) x (1, 0, 0) in component "06_Sottoassieme_coperchio_stepper_torretta"
  line L0 (-20, 0) -> (20, 0)
component "01_Piano_inferiore_colonnine_M3_supporto_batteria_integrato" placed x (1, 0, 0) y (0, 1, 0) z (0, 0, 1) at (0, 0, 0)
component "02_Piano_superiore" placed x (1, 0, 0) y (0, 1, 0) z (0, 0, 1) at (0, 0, 0)
component "03_Guscio_laterale_continuo_carro" placed x (1, 0, 0) y (0, 1, 0) z (0, 0, 1) at (0, 0, 0)
component "05_Arduino_UNO_R4_WiFi_RIFERIMENTO_XY_quota_Z_da_definire" placed x (1, 0, 0) y (0, 1, 0) z (0, 0, 1) at (33.33, 45.71, 3)
component "06_Sottoassieme_coperchio_stepper_torretta" placed x (1, 0, 0) y (0, 1, 0) z (0, 0, 1) at (0, 0, 46)
component "01_Tetto_elettronica_removibile" placed x (1, 0, 0) y (0, 1, 0) z (0, 0, 1) at (0, 0, 0) in component "06_Sottoassieme_coperchio_stepper_torretta"
component "02A_Rondella_assiale_torretta_sostituibile" placed x (1, 0, 0) y (0, 1, 0) z (0, 0, 1) at (0, 0, 0) in component "06_Sottoassieme_coperchio_stepper_torretta"
component "02_Stepper_28BYJ48_statore_fisso_riferimento" placed x (1, 0, 0) y (0, 1, 0) z (0, 0, 1) at (0, 0, 0) in component "06_Sottoassieme_coperchio_stepper_torretta"
component "02B_Rotore_albero_28BYJ48_riferimento" placed x (1, 0, 0) y (0, 1, 0) z (0, 0, 1) at (0, 0, 0) in component "06_Sottoassieme_coperchio_stepper_torretta"
component "03_Base_rotante_D100_sede_D_stepper" placed x (1, 0, 0) y (0, 1, 0) z (0, 0, 1) at (0, 0, 0) in component "06_Sottoassieme_coperchio_stepper_torretta"
component "03A_Fermaglio_anti_sollevamento_Est_M3" placed x (1, 0, 0) y (0, 1, 0) z (0, 0, 1) at (0, 0, 0) in component "06_Sottoassieme_coperchio_stepper_torretta"
component "03A_Fermaglio_anti_sollevamento_Ovest_M3" placed x (1, 0, 0) y (0, 1, 0) z (0, 0, 1) at (0, 0, 0) in component "06_Sottoassieme_coperchio_stepper_torretta"
component "03A_Fermaglio_anti_sollevamento_Nord_M3" placed x (1, 0, 0) y (0, 1, 0) z (0, 0, 1) at (0, 0, 0) in component "06_Sottoassieme_coperchio_stepper_torretta"
component "03A_Fermaglio_anti_sollevamento_Sud_M3" placed x (1, 0, 0) y (0, 1, 0) z (0, 0, 1) at (0, 0, 0) in component "06_Sottoassieme_coperchio_stepper_torretta"
component "04_Torretta_parte_fissa_azimut" placed x (1, 0, 0) y (0, 1, 0) z (0, 0, 1) at (0, 0, 0) in component "06_Sottoassieme_coperchio_stepper_torretta"
component "05_Servo_TowerPro_SG90_Sinistro_statore_riferimento" placed x (1, 0, 0) y (0, 1, 0) z (0, 0, 1) at (0, 0, 0) in component "06_Sottoassieme_coperchio_stepper_torretta"
component "06_Servo_TowerPro_SG90_Destro_statore_riferimento" placed x (1, 0, 0) y (0, 1, 0) z (0, 0, 1) at (0, 0, 0) in component "06_Sottoassieme_coperchio_stepper_torretta"
component "09_Torretta_parte_mobile_elevazione" placed x (1, 0, 0) y (0, 1, 0) z (0, 0, 1) at (0, 0, 0) in component "06_Sottoassieme_coperchio_stepper_torretta"
component "07_Albero_e_cornetto_croce_SG90_Sinistro_riferimento" placed x (1, 0, 0) y (0, 1, 0) z (0, 0, 1) at (0, 0, 0) in component "06_Sottoassieme_coperchio_stepper_torretta"
component "08_Albero_e_cornetto_croce_SG90_Destro_riferimento" placed x (1, 0, 0) y (0, 1, 0) z (0, 0, 1) at (0, 0, 0) in component "06_Sottoassieme_coperchio_stepper_torretta"
component "09A_Guancia_cornetto_Sinistra_regolabile" placed x (1, 0, 0) y (0, 1, 0) z (0, 0, 1) at (0, 0, 0) in component "06_Sottoassieme_coperchio_stepper_torretta"
component "09B_Guancia_cornetto_Destra_regolabile" placed x (1, 0, 0) y (0, 1, 0) z (0, 0, 1) at (0, 0, 0) in component "06_Sottoassieme_coperchio_stepper_torretta"
component "10_Modulo_cannone_reale_PCB_solenoide_canna" placed x (1, 0, 0) y (0, 1, 0) z (0, 0, 1) at (0, 0, 0) in component "06_Sottoassieme_coperchio_stepper_torretta"
component "11_Guscio_fisso_posteriore_torretta_removibile" placed x (1, 0, 0) y (0, 1, 0) z (0, 0, 1) at (0, 0, 0) in component "06_Sottoassieme_coperchio_stepper_torretta"
component "12_Carter_SG90_Sinistro_removibile" placed x (1, 0, 0) y (0, 1, 0) z (0, 0, 1) at (0, 0, 0) in component "06_Sottoassieme_coperchio_stepper_torretta"
component "13_Carter_SG90_Destro_removibile" placed x (1, 0, 0) y (0, 1, 0) z (0, 0, 1) at (0, 0, 0) in component "06_Sottoassieme_coperchio_stepper_torretta"
component "14_Guscio_mobile_cannone_removibile" placed x (1, 0, 0) y (0, 1, 0) z (0, 0, 1) at (0, 0, 0) in component "06_Sottoassieme_coperchio_stepper_torretta"
component "15_Coperchio_culatta_L_removibile_M2_5" placed x (1, 0, 0) y (0, 1, 0) z (0, 0, 1) at (0, 0, 0) in component "06_Sottoassieme_coperchio_stepper_torretta"
equation "piano_inf_lunghezza = 170.0 mm" comment "Piano inferiore"
equation "piano_inf_larghezza = 160.0 mm" comment "Piano inferiore"
equation "piano_inf_spessore = 3.0 mm" comment "Piano inferiore"
equation "d4 = piano_inf_spessore"
equation "distanza_piani = 40.0 mm" comment "Luce libera fra i piani"
equation "piano_sup_lunghezza = 170.0 mm" comment "Piano superiore"
equation "piano_sup_larghezza = 160.0 mm" comment "Piano superiore"
equation "piano_sup_spessore = 3.0 mm" comment "Piano superiore"
equation "colonnina_diametro = 10.0 mm" comment "Colonnine base"
equation "foro_vite_M3 = 3.2 mm" comment "Gioco vite M3"
equation "colonnina_offset_bordo = 12.0 mm" comment "Centro colonnina dal bordo"
equation "dado_M3_chiave = 5.8 mm" comment "Sede esagonale dado M3"
equation "dado_M3_profondita = 2.6 mm" comment "Profondita sede dado M3"
equation "d15 = piano_inf_spessore + distanza_piani"
equation "d17 = piano_sup_spessore"
equation "d19 = piano_inf_spessore"
equation "d21 = piano_inf_spessore + distanza_piani - dado_M3_profondita"
equation "asola_fascetta_lunghezza = 10.0 mm" comment "Asola fascetta, asse Est-Ovest"
equation "asola_fascetta_larghezza = 5.0 mm" comment "Asola fascetta, asse Sud-Nord"
equation "d25 = piano_inf_spessore"
equation "d27 = piano_inf_spessore"
equation "d29 = piano_inf_spessore"
equation "d31 = piano_inf_spessore"
equation "foro_servizio_inferiore_larghezza = 10.0 mm" comment "Foro 10x10 vicino Arduino"
equation "foro_servizio_inferiore_lunghezza = 10.0 mm" comment "Foro 10x10 vicino Arduino"
equation "foro_servizio_inferiore_centro_x = -0.5 mm" comment "Centro quasi sull'asse del carro"
equation "foro_servizio_inferiore_da_sud = 110.0 mm" comment "20 mm oltre il centro dell'ultima asola fascetta"
equation "d37 = piano_inf_spessore"
equation "d39 = piano_sup_spessore"
equation "d41 = distanza_piani"
equation "d43 = piano_inf_spessore + distanza_piani"
equation "d45 = dado_M3_profondita"
equation "d47 = piano_sup_spessore"
equation "d49 = distanza_piani"
equation "d51 = piano_inf_spessore + distanza_piani"
equation "d53 = dado_M3_profondita"
equation "d55 = piano_sup_spessore"
equation "d57 = distanza_piani"
equation "d59 = piano_inf_spessore + distanza_piani"
equation "d61 = dado_M3_profondita"
equation "d63 = piano_sup_spessore"
equation "d65 = distanza_piani"
equation "d67 = piano_inf_spessore + distanza_piani"
equation "d69 = dado_M3_profondita"
equation "apertura_arduino_larghezza = 25.0 mm" comment "Apertura superiore sopra Arduino"
equation "apertura_arduino_lunghezza = 25.0 mm" comment "Apertura superiore sopra Arduino"
equation "apertura_arduino_centro_x = 33.33 mm" comment "Centro Est-Ovest apertura Arduino"
equation "apertura_arduino_centro_y = 45.71 mm" comment "Centro Sud-Nord apertura Arduino"
equation "apertura_pacco_batteria_larghezza = 33.0 mm" comment "Apertura superiore pacco batteria PCB cannone"
equation "apertura_pacco_batteria_lunghezza = 60.0 mm" comment "Apertura superiore pacco batteria PCB cannone"
equation "apertura_pacco_batteria_centro_x = -52.5 mm" comment "Centro Est-Ovest apertura pacco batteria PCB cannone"
equation "apertura_pacco_batteria_centro_y = -15.0 mm" comment "Centro Sud-Nord apertura pacco batteria PCB cannone"
equation "d79 = piano_sup_spessore"
equation "d81 = piano_sup_spessore"
equation "foro_piano_superiore_M2_5_guscio = 2.7 mm" comment "Quattro viti M2.5x8 per trattenere il guscio inferiore"
equation "d84 = piano_sup_spessore"
equation "d86 = piano_sup_spessore"
equation "d88 = piano_sup_spessore"
equation "d90 = piano_sup_spessore"
equation "batt_vano_lunghezza = 95.0 mm" comment "Vano batteria"
equation "batt_vano_larghezza = 40.0 mm" comment "Vano batteria"
equation "batt_esterno_lunghezza = 100.0 mm" comment "Supporto batteria"
equation "batt_esterno_larghezza = 45.0 mm" comment "Supporto batteria"
equation "batt_parete_spessore = 2.5 mm" comment "Pareti laterali"
equation "batt_parete_altezza = 17.0 mm" comment "Pareti laterali"
equation "batt_apertura_cavi = 10.0 mm" comment "Passaggio cavi"
equation "d99 = piano_inf_spessore"
equation "d101 = batt_parete_altezza"
equation "d103 = batt_parete_altezza"
equation "d105 = batt_parete_altezza"
equation "d107 = batt_parete_altezza"
equation "guscio_carro_larghezza_interna = 161.0 mm" comment "Vano interno guscio carro"
equation "guscio_carro_lunghezza_interna = 171.0 mm" comment "Vano interno guscio carro"
equation "guscio_carro_larghezza_esterna = 166.0 mm" comment "Ingombro esterno guscio carro"
equation "guscio_carro_lunghezza_esterna = 176.0 mm" comment "Ingombro esterno guscio carro"
equation "guscio_carro_parete = 2.5 mm" comment "Pareti guscio removibile"
equation "guscio_carro_altezza_inferiore = 46.0 mm" comment "Da piano inferiore a sommità piano superiore"
equation "guscio_carro_gioco_lato = 0.5 mm" comment "Gioco per lato rispetto ai piani"
equation "guscio_carro_altezza_laterale_continua = 76.0 mm" comment "Parete unica senza giunzione intermedia"
equation "guscio_linguetta_M2_5_spessore = 5.0 mm" comment "Fissaggio guscio sotto il piano superiore"
equation "guscio_linguetta_M2_5_span = 14.0 mm" comment "Fissaggio guscio sotto il piano superiore"
equation "guscio_linguetta_M2_5_profondita = 13.0 mm" comment "Fissaggio guscio sotto il piano superiore"
equation "guscio_linguetta_M2_5_preforo = 2.2 mm" comment "Preforo per M2.5x8"
equation "griglia_feritoie_per_parete = 3.0 mm" comment "Numero ridotto di feritoie fronte e retro"
equation "griglia_feritoia_larghezza = 42.0 mm" comment "Ventilazione vano inferiore"
equation "griglia_feritoia_altezza = 4.0 mm" comment "Ventilazione vano inferiore"
equation "griglia_feritoia_passo_verticale = 8.0 mm" comment "Ventilazione vano inferiore"
equation "d125 = guscio_carro_altezza_laterale_continua"
equation "d127 = guscio_carro_altezza_laterale_continua"
equation "d129 = guscio_carro_altezza_laterale_continua"
equation "d131 = guscio_carro_altezza_laterale_continua"
equation "arduino_r4_lunghezza = 68.58 mm" comment "Profilo ufficiale Arduino UNO R4 WiFi"
equation "arduino_r4_larghezza = 53.34 mm" comment "Profilo ufficiale Arduino UNO R4 WiFi"
equation "arduino_r4_spessore_pcb = 1.0 mm" comment "Spessore PCB ufficiale; quota Z di montaggio non ancora definita"
equation "arduino_r4_rotazione = 90.0 deg" comment "Jack DC orientato verso Sud"
equation "arduino_r4_centro_x = 33.33 mm" comment "Posizione planimetrica Arduino"
equation "arduino_r4_centro_y = 45.71 mm" comment "Posizione planimetrica Arduino"
equation "cop_lunghezza = 176.0 mm" comment "Ingombro coperchio"
equation "cop_larghezza = 166.0 mm" comment "Ingombro coperchio"
equation "cop_parete_altezza = 30.0 mm" comment "Quota locale del tetto removibile"
equation "cop_tetto_spessore = 3.0 mm" comment "Coperchio elettronica"
equation "cop_boss_M3_diametro = 10.0 mm" comment "Accesso vite M3 dal tetto alle colonnine"
equation "cop_canale_fondo_raggio_interno = 19.0 mm" comment "Fondo liscio pista cavi tipo clock-spring"
equation "cop_canale_fondo_raggio_esterno = 40.0 mm" comment "Fondo liscio pista cavi tipo clock-spring"
equation "cop_canale_fondo_quota = 20.0 mm" comment "Quota locale fondo pista cavi"
equation "cop_canale_fondo_spessore = 3.0 mm" comment "Fondo strutturale pista cavi"
equation "cop_canale_parete_spessore = 1.5 mm" comment "Pareti lisce pista cavi"
equation "cop_canale_altezza_libera = 7.0 mm" comment "Altezza libera pista cavi"
equation "stepper_corpo_diametro = 28.0 mm" comment "Riferimento stepper"
equation "stepper_corpo_altezza = 20.0 mm" comment "Riferimento stepper"
equation "stepper_albero_diametro = 5.0 mm" comment "Riferimento stepper"
equation "stepper_albero_quota_piatto = 3.0 mm" comment "Profilo D confermato"
equation "stepper_albero_lunghezza = 9.0 mm" comment "Riferimento stepper"
equation "stepper_interasse_fori = 35.0 mm" comment "Fissaggio stepper"
equation "stepper_foro_fissaggio = 4.2 mm" comment "Fissaggio stepper"
equation "stepper_svasatura_M4_diametro = 8.4 mm" comment "Testa svasata a filo"
equation "stepper_svasatura_M4_profondita = 2.1 mm" comment "Testa svasata a filo"
equation "torre_base_diametro = 100.0 mm" comment "Adattatore rotante"
equation "torre_base_spessore = 6.0 mm" comment "Adattatore rotante"
equation "torre_sede_D_diametro = 5.4 mm" comment "Mozzo D stepper"
equation "torre_sede_D_quota_piatto = 3.2 mm" comment "Mozzo D stepper"
equation "torre_rondella_assiale_DI = 76.0 mm" comment "Appoggio assiale esterno ai cavi"
equation "torre_rondella_assiale_DE = 94.0 mm" comment "Appoggio assiale esterno ai cavi"
equation "torre_rondella_assiale_spessore = 0.8 mm" comment "Appoggio assiale esterno ai cavi"
equation "torre_rondella_sede_profondita = 0.3 mm" comment "Localizzazione rondella"
equation "torre_rondella_sede_gioco = 0.2 mm" comment "Gioco per lato sede rondella"
equation "torre_guida_fissa_RI = 34.5 mm" comment "Centraggio radiale"
equation "torre_guida_fissa_RE = 36.5 mm" comment "Centraggio radiale"
equation "torre_guida_fissa_altezza = 2.6 mm" comment "Centraggio radiale"
equation "torre_gola_gioco_radiale = 0.3 mm" comment "Gioco per lato"
equation "torre_gola_profondita = 2.5 mm" comment "Guida rotante"
equation "torre_fermaglio_gioco_verticale = 0.4 mm" comment "Anti-sollevamento"
equation "torre_fermaglio_sovrapposizione = 1.5 mm" comment "Anti-sollevamento"
equation "torre_fermaglio_foro_M3 = 3.2 mm" comment "Fermagli removibili"
equation "torre_fermaglio_spallamento_altezza = 1.5 mm" comment "Antirotazione fermagli"
equation "torre_fermaglio_spallamento_larghezza = 2.0 mm" comment "Antirotazione fermagli"
equation "torre_distanziale_telaio_altezza = 6.0 mm" comment "Evita collisione con fermagli"
equation "torre_distanziale_telaio_diametro = 10.0 mm" comment "Quattro appoggi M3"
equation "torre_fissa_larghezza = 80.0 mm" comment "Parte fissa torretta"
equation "torre_fissa_lunghezza = 70.0 mm" comment "Parte fissa torretta"
equation "torre_fissa_altezza = 50.0 mm" comment "Parte fissa torretta"
equation "torre_parete_spessore = 4.0 mm" comment "Parte fissa torretta"
equation "torre_perno_quota = 32.0 mm" comment "Asse elevazione"
equation "servo_corpo_lunghezza = 22.7 mm" comment "TowerPro SG90"
equation "servo_corpo_larghezza = 12.2 mm" comment "TowerPro SG90"
equation "servo_corpo_altezza = 27.0 mm" comment "TowerPro SG90"
equation "servo_ingombro_con_uscita = 30.3 mm" comment "TowerPro SG90"
equation "servo_alette_lunghezza_totale = 32.3 mm" comment "TowerPro SG90"
equation "servo_aletta_sporgenza = 5.0 mm" comment "Quota utente circa 5 mm"
equation "servo_aletta_spessore = 2.0 mm" comment "Quota utente 2 mm"
equation "servo_aletta_foro_M2_5 = 2.5 mm" comment "M2.5 provata sul pezzo"
equation "servo_aletta_asola_telaio_lunghezza = 5.0 mm" comment "Registrazione lungo Y"
equation "servo_aletta_asola_telaio_larghezza = 2.9 mm" comment "Passaggio M2.5 con gioco"
equation "servo_aletta_parete_minima = 1.2 mm" comment "Tra asola e finestra corpo"
equation "servo_asse_da_estremita = 17.0 mm" comment "TowerPro SG90"
equation "servo_albero_sporgenza = 3.3 mm" comment "TowerPro SG90"
equation "servo_albero_diametro_riferimento = 6.0 mm" comment "Solo inviluppo uscita SG90"
equation "servo_cornetto_span_riferimento = 33.0 mm" comment "Cornetto reale usato come dima"
equation "servo_cornetto_spessore_riferimento = 1.5 mm" comment "Quota visiva provvisoria"
equation "servo_adattatore_cornetto_diametro = 34.0 mm" comment "Disco pieno senza interassi inventati"
equation "servo_adattatore_cornetto_spessore = 4.0 mm" comment "Impegno viti appuntite"
equation "servo_adattatore_accesso_vite_centrale = 10.0 mm" comment "Accesso alla vite originale"
equation "servo_adattatore_asola_regolazione = 5.0 mm" comment "Registrazione assiale"
equation "servo_gioco_inserimento = 0.5 mm" comment "Slitta servo"
equation "servo_supporto_parete = 2.5 mm" comment "Slitta servo"
equation "servo_supporto_ripiano = 2.5 mm" comment "Slitta servo"
equation "servo_carter_foro_M2_5 = 2.7 mm" comment "Carter removibile"
equation "servo_carter_preforo_M2_5 = 2.2 mm" comment "Supporto carter"
equation "servo_cavo_larghezza = 4.0 mm" comment "Cavo piatto SG90"
equation "servo_cavo_spessore = 1.0 mm" comment "Cavo piatto SG90"
equation "servo_uscita_cavo_larghezza = 5.0 mm" comment "Slitta SG90"
equation "servo_uscita_cavo_profondita = 2.0 mm" comment "Slitta SG90"